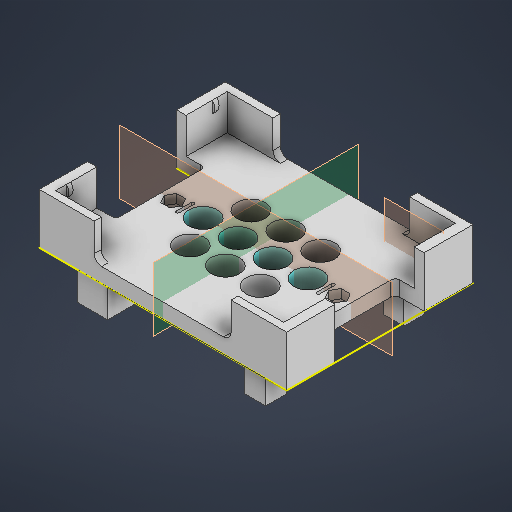
# Autodesk Inventor part: PILLARSCELLCASE18650
Saved by Autodesk Inventor 2026.2 (Build 302298000, 298)
## iProperties
Created: 2024-11-21
Part Number: PILLARSCELLCASE18650
Material: Generic
Document SubType Name: Modeling
Designer: cbast
Density: 1 g/cm^3
Appearance: Default
Mass: 190.937 g
Surface Area: 666.623 cm^2
Volume: 190.937 cm^3
Author: cbast
## iProperties of the stored document BatteryCasev1_3DPrint.ipt
Created: 2025-01-30
Part Number: BatteryCasev1_3DPrint
Material: Generic
Document SubType Name: Modeling
Designer: cbast
Density: 1 g/cm^3
Appearance: Default
Author: cbast
Autodesk Inventor part; units mm, degrees
ref_plane "YZ Plane" through (0, 0, 0) normal (1, 0, 0) x (0, 1, 0)
ref_plane "XZ Plane" through (0, 0, 0) normal (0, 1, 0) x (-1, 0, 0)
ref_plane "XY Plane" through (0, 0, 0) normal (0, 0, 1) x (1, 0, 0)
sketch "Sketch1" plane through (0, 0, 0) normal (0, 1, 0) x (-1, 0, 0)
  circle A0 centre (0, 0) radius 9.5
  circle A1 centre (23.5, 0) radius 9.5
  circle A2 centre (-23.5, 0) radius 9.5
  circle A3 centre (47, 0) radius 9.5
  line L0 (0, 0) -> (-32.9562, 0) construction
  line L1 (-32.9562, 0) -> (61.076, 0) construction
  circle A4 centre (0, 0) radius 14 construction
  circle A5 centre (-23.5, 0) radius 14 construction
  circle A6 centre (47, 0) radius 14 construction
  circle A7 centre (23.5, 0) radius 14 construction
  circle A8 centre (47, 0) radius 15 construction
  circle A9 centre (-23.5, 0) radius 15 construction
  circle A10 centre (0, 0) radius 15 construction
  circle A11 centre (23.5, 0) radius 15 construction
  line L2 (37.5, 0) -> (33, 0) construction
  circle A12 centre (35.25, -20.3516) radius 9.5
  circle A13 centre (35.25, -20.3516) radius 14 construction
  circle A14 centre (35.25, -20.3516) radius 15 construction
  line L3 (14, 0) -> (9.5, 0) construction
  line L4 (-9.5, 0) -> (-14, 0) construction
  line L5 (35.25, -20.3516) -> (-11.75, -20.3516) construction
  circle A15 centre (11.75, -20.3516) radius 9.5
  circle A16 centre (-11.75, -20.3516) radius 9.5
  circle A17 centre (11.75, -20.3516) radius 14 construction
  circle A18 centre (11.75, -20.3516) radius 15 construction
  circle A19 centre (-11.75, -20.3516) radius 14 construction
  circle A20 centre (-11.75, -20.3516) radius 15 construction
  circle A21 centre (35.25, 20.3516) radius 9.5
  circle A22 centre (35.25, 20.3516) radius 14 construction
  circle A23 centre (35.25, 20.3516) radius 15 construction
  line L6 (35.25, 20.3516) -> (-11.75, 20.3516) construction
  circle A24 centre (11.75, 20.3516) radius 9.5
  circle A25 centre (-11.75, 20.3516) radius 9.5
  circle A26 centre (11.75, 20.3516) radius 14 construction
  circle A27 centre (11.75, 20.3516) radius 15 construction
  circle A28 centre (-11.75, 20.3516) radius 14 construction
  circle A29 centre (-11.75, 20.3516) radius 15 construction
  arc A30 (49.1998, -14.8378) -> (49.1998, 14.8378) centre (47, 0) ccw
  arc A31 (49.1998, 14.8378) -> (23.5, 29.6756) centre (35.25, 20.3516) ccw
  arc A32 (23.5, 29.6756) -> (0, 29.6756) centre (11.75, 20.3516) ccw
  arc A33 (0, 29.6756) -> (-25.6998, 14.8378) centre (-11.75, 20.3516) ccw
  arc A34 (-25.6998, 14.8378) -> (-25.6998, -14.8378) centre (-23.5, 0) ccw
  arc A35 (-25.6998, -14.8378) -> (0, -29.6756) centre (-11.75, -20.3516) ccw
  arc A36 (0, -29.6756) -> (23.5, -29.6756) centre (11.75, -20.3516) ccw
  arc A37 (23.5, -29.6756) -> (49.1998, -14.8378) centre (35.25, -20.3516) ccw
  point P0 (46.8931, -14.9996)
  point P1 (46.8931, 14.9996)
  point P2 (-23.3931, 14.9996)
  point P3 (-23.3931, -14.9996)
  dimension "d145" = 28
  dimension "d149" = 28
  dimension "d0" = 19
  dimension "d2" = 19
  dimension "d4" = 19
  dimension "d53" = 19
  dimension "d144" = 28
  dimension "d150" = 28
  dimension "d154" = 30
  dimension "d158" = 30
  dimension "d162" = 30
  dimension "d163" = 30
  dimension "d291" = 19
  dimension "d292" = 28
  dimension "d293" = 30
  dimension "d294" = 19
  dimension "d295" = 19
  dimension "d296" = 28
  dimension "d297" = 30
  dimension "d298" = 28
  dimension "d299" = 30
  constraints: 40 point on circle, 36 centre point, 32 coincident, 12 end point, 10 vertical alignment, 9 equal radius, 4 tangent, 2 horizontal alignment, 1 horizontal, 1 midpoint, 1 parallel, 1 point on line, 17 other
  measures "d0" diameter of A0
  measures "d2" diameter of A1
  measures "d4" diameter of A2
  measures "d53" diameter of A3
  measures "d144" diameter of A4
  measures "d150" diameter of A7
  measures "d154" diameter of A8
  measures "d158" diameter of A9
  measures "d162" diameter of A10
  measures "d163" diameter of A11
  measures "d291" diameter of A12
  measures "d292" diameter of A13
  measures "d293" diameter of A14
  measures "d294" diameter of A15
  measures "d295" diameter of A16
  measures "d296" diameter of A17
  measures "d297" diameter of A18
  measures "d298" diameter of A19
  measures "d299" diameter of A20
extrude "Extrusion1" add sketch "Sketch1" along normal blind 15
sketch "Sketch26" plane through (0, 15, 0) normal (0, 1, 0) x (1, 0, 0)
  arc A0 (-49.1998, -14.8378) -> (-23.5, -29.6756) centre (-35.25, -20.3516) ccw projected
  arc A1 (-23.5, -29.6756) -> (0, -29.6756) centre (-11.75, -20.3516) ccw projected
  arc A2 (0, -29.6756) -> (25.6998, -14.8378) centre (11.75, -20.3516) ccw projected
  arc A3 (25.6998, -14.8378) -> (25.6998, 14.8378) centre (23.5, 0) ccw projected
  arc A4 (25.6998, 14.8378) -> (0, 29.6756) centre (11.75, 20.3516) ccw projected
  arc A5 (0, 29.6756) -> (-23.5, 29.6756) centre (-11.75, 20.3516) ccw projected
  arc A6 (-23.5, 29.6756) -> (-49.1998, 14.8378) centre (-35.25, 20.3516) ccw projected
  arc A7 (-49.1998, 14.8378) -> (-49.1998, -14.8378) centre (-47, 0) ccw projected
  circle A8 centre (0, 0) radius 9.5 projected
  circle A9 centre (-23.5, 0) radius 9.5 projected
  circle A10 centre (11.75, -20.3516) radius 9.5 projected
  circle A11 centre (-11.75, -20.3516) radius 9.5 projected
  circle A12 centre (-35.25, -20.3516) radius 9.5 projected
  circle A13 centre (11.75, 20.3516) radius 9.5 projected
  circle A14 centre (-11.75, 20.3516) radius 9.5 projected
  circle A15 centre (-35.25, 20.3516) radius 9.5 projected
  circle A16 centre (-47, 0) radius 9.5 projected
  circle A17 centre (23.5, 0) radius 9.5 projected
  line L0 (-88.45, 57.7) -> (64.95, 57.7)
  line L1 (64.95, 57.7) -> (64.95, -57.7)
  line L2 (64.95, -57.7) -> (-88.45, -57.7)
  line L3 (-88.45, -57.7) -> (-88.45, 57.7)
  line L4 (-88.45, 57.7) -> (64.95, -57.7) construction
  line L5 (64.95, 57.7) -> (-88.45, -57.7) construction
  line L6 (-88.45, 0) -> (-62, 0) construction
  line L7 (38.5, 0) -> (64.95, 0) construction
  point P0 (-11.75, 0)
  dimension "d300" = 153.4
  dimension "d301" = 115.4
  constraints: 16 end point, 4 midpoint, 3 equal length, 2 horizontal, 2 point on circle, 1 collinear, 1 perpendicular
  measures "d300" distance of L1.end L2.end
  measures "d301" distance of L0.end L1.end
extrude "Extrusion24" add sketch "Sketch26" against normal blind 10 contours L0 L1 L2 L3
sketch "Sketch28" plane through (0, 15, 0) normal (0, 1, 0) x (1, 0, 0)
  line L0 (-88.45, -57.7) -> (64.95, -57.7) projected
  line L1 (64.95, -57.7) -> (64.95, 57.7) projected
  line L2 (64.95, 57.7) -> (-88.45, 57.7) projected
  line L3 (-88.45, 57.7) -> (-88.45, -57.7) projected
  circle A0 centre (0, 0) radius 9.5 projected
  circle A1 centre (-23.5, 0) radius 9.5 projected
  circle A2 centre (11.75, -20.3516) radius 9.5 projected
  circle A3 centre (-11.75, -20.3516) radius 9.5 projected
  circle A4 centre (-35.25, -20.3516) radius 9.5 projected
  circle A5 centre (11.75, 20.3516) radius 9.5 projected
  circle A6 centre (-11.75, 20.3516) radius 9.5 projected
  circle A7 centre (-35.25, 20.3516) radius 9.5 projected
  circle A8 centre (-47, 0) radius 9.5 projected
  circle A9 centre (23.5, 0) radius 9.5 projected
  line L4 (64.95, 57.7) -> (64.95, -57.7) projected
  line L5 (-88.0641, -57.4308) -> (64.95, -57.4308)
  line L6 (64.95, -57.4308) -> (64.95, 57.7)
  line L7 (64.95, 57.7) -> (-88.0641, 57.7)
  line L8 (-88.0641, 57.7) -> (-88.0641, -57.4308)
  line L9 (-88.0641, -57.4308) -> (64.95, 57.7) construction
  line L10 (64.95, -57.4308) -> (-88.0641, 57.7) construction
  line L11 (-94.7093, -62.4308) -> (71.5952, -62.4308)
  line L12 (71.5952, -62.4308) -> (71.5952, 62.7)
  line L13 (71.5952, 62.7) -> (-94.7093, 62.7)
  line L14 (-94.7093, 62.7) -> (-94.7093, -62.4308)
  line L15 (-94.7093, -62.4308) -> (71.5952, 62.7) construction
  line L16 (71.5952, -62.4308) -> (-94.7093, 62.7) construction
  point P0 (-11.5571, 0.1346)
  point P1 (-11.5571, 0.1346)
  dimension "d306" = 5
  constraints: 24 end point, 5 midpoint, 4 parallel, 2 horizontal, 2 perpendicular, 1 point on line
  measures "d306" distance between parallel lines of L13 L2
extrude "Extrusion25" add sketch "Sketch28" along normal blind 24 and the other way blind 10 contours L14 L13 L12 L11
sketch "Sketch29" plane through (-94.7093, 39, 62.4308) normal (0, 0, 1) x (1, 0, 0)
  line L0 (6.2593, -24) -> (159.6593, -24) projected
  line L1 (41.9593, -24) -> (123.9593, -24)
  line L2 (166.3046, 0) -> (0, 0) projected
  line L3 (128.9593, -24) -> (36.9593, -24)
  line L4 (36.9593, -19) -> (36.9593, 0)
  line L5 (36.9593, 0) -> (128.9593, 0)
  line L6 (128.9593, 0) -> (128.9593, -19)
  arc A0 (36.9593, -19) -> (41.9593, -24) centre (41.9593, -19) ccw
  arc A1 (123.9593, -24) -> (128.9593, -19) centre (123.9593, -19) ccw
  point P0 (94.7093, -39)
  point P1 (82.9593, -24)
  point P2 (42.9593, -24)
  point P3 (128.9593, 0)
  dimension "d311" = 86
  dimension "d312" = 5
  constraints: 10 end point, 6 point on line, 4 point on circle, 4 tangent, 2 centre point, 2 midpoint, 2 parallel, 1 equal radius, 1 horizontal, 1 perpendicular
  measures "d311" distance of point (42.959, -24) L3.start
  measures "d312" radius of A0
extrude "Extrusion26" cut sketch "Sketch29" against normal through all
sketch "Sketch30" plane through (0, 39, 0) normal (0, 1, 0) x (1, 0, 0)
  circle A0 centre (-47, 0) radius 9.5 projected
  circle A1 centre (0, 0) radius 9.5 projected
  circle A2 centre (-23.5, 0) radius 9.5 projected
  circle A3 centre (11.75, -20.3516) radius 9.5 projected
  circle A4 centre (-11.75, -20.3516) radius 9.5 projected
  circle A5 centre (-35.25, -20.3516) radius 9.5 projected
  circle A6 centre (11.75, 20.3516) radius 9.5 projected
  circle A7 centre (-11.75, 20.3516) radius 9.5 projected
  circle A8 centre (-35.25, 20.3516) radius 9.5 projected
  circle A9 centre (23.5, 0) radius 9.5 projected
  line L0 (29.25, -57.7) -> (64.95, -57.7) projected
  line L1 (64.95, -57.7) -> (64.95, 57.7) projected
  line L2 (64.95, 57.7) -> (29.25, 57.7) projected
  line L3 (29.25, 57.7) -> (29.25, 62.7) projected
  line L4 (-52.75, 62.7) -> (29.25, 62.7) projected
  line L5 (-52.75, 57.7) -> (-52.75, 62.7) projected
  line L6 (-52.75, 57.7) -> (-88.45, 57.7) projected
  line L7 (-88.45, 57.7) -> (-88.45, -57.7) projected
  line L8 (-88.45, -57.7) -> (-52.75, -57.7) projected
  line L9 (-52.75, -62.4308) -> (-52.75, -57.7) projected
  line L10 (29.25, -62.4308) -> (-52.75, -62.4308) projected
  line L11 (29.25, -62.4308) -> (29.25, -57.7) projected
  line L12 (34.25, -57.7) -> (34.25, -62.4308) projected
  line L13 (34.25, -62.4308) -> (71.5952, -62.4308) projected
  line L14 (71.5952, -62.4308) -> (71.5952, 62.7) projected
  line L15 (71.5952, 62.7) -> (34.25, 62.7) projected
  line L16 (34.25, 62.7) -> (34.25, 57.7) projected
  line L17 (34.25, 57.7) -> (64.95, 57.7) projected
  line L18 (64.95, 57.7) -> (64.95, -57.7) projected
  line L19 (64.95, -57.7) -> (34.25, -57.7) projected
  line L20 (-88.45, -57.7) -> (-88.45, 57.7) projected
  line L21 (-57.75, -62.4308) -> (-57.75, -57.7) projected
  line L22 (-57.75, -57.7) -> (-88.45, -57.7) projected
  line L23 (-88.45, -57.7) -> (-88.45, 57.7) projected
  line L24 (-88.45, 57.7) -> (-57.75, 57.7) projected
  line L25 (-57.75, 57.7) -> (-57.75, 62.7) projected
  line L26 (-57.75, 62.7) -> (-94.7093, 62.7) projected
  line L27 (-94.7093, 62.7) -> (-94.7093, -62.4308) projected
  line L28 (-94.7093, -62.4308) -> (-57.75, -62.4308) projected
  line L29 (-88.45, -30) -> (-88.45, 30)
  line L30 (-94.7093, -62.4308) -> (-94.7093, 62.7) projected
  line L31 (-75.7093, 27) -> (-75.7093, -27)
  arc A10 (-75.7093, 27) -> (-78.7093, 30) centre (-78.7093, 27) ccw
  arc A11 (-78.7093, -30) -> (-75.7093, -27) centre (-78.7093, -27) ccw
  line L32 (-94.7093, 0) -> (-47, 0) construction
  line L33 (-47, 0) -> (-94.7093, 0) construction
  line L34 (-78.7093, 30) -> (-114.521, 30)
  line L35 (-114.521, 30) -> (-114.521, -30)
  line L36 (-114.521, -30) -> (-78.7093, -30)
  point P0 (-88.45, 0)
  dimension "d317" = 3
  constraints: 14 end point, 4 point on circle, 3 perpendicular, 2 centre point, 2 midpoint, 2 tangent, 1 collinear, 1 equal radius, 1 horizontal
  measures "d317" radius of A10
extrude "Extrusion27" cut sketch "Sketch30" against normal through all contours L36 L27 L34 L7 | L7 L34 A10 L31 A11 L36 | L36 L35 L34 L27
ref_plane "Work Plane9" through (-11.75, 15, -57.7) normal (-1, 0, 0) x (0, 0, 1)
sketch "Sketch31" plane through (0, 15, 0) normal (0, 1, 0) x (1, 0, 0)
  line L0 (-64.06, 5.3) -> (-61, 0)
  line L1 (-61, 0) -> (-64.06, -5.3)
  line L2 (-64.06, -5.3) -> (-70.1799, -5.3)
  line L3 (-70.1799, -5.3) -> (-73.2398, 0)
  line L4 (-73.2398, 0) -> (-70.1799, 5.3)
  line L5 (-70.1799, 5.3) -> (-64.06, 5.3)
  line L6 (-88.45, 57.7) -> (-57.75, 57.7) projected
  circle A0 centre (-47, 0) radius 9.5 projected
  line L7 (-57.75, -57.7) -> (-88.45, -57.7) projected
  line L8 (-75.7093, -27) -> (-75.7093, 27) construction
  line L9 (-75.7093, 0) -> (-47, 0) construction
  point P0 (0, 0)
  point P1 (-67.1199, 0)
  dimension "d323" = 14
  dimension "d332" = 10.6
  constraints: 14 end point, 2 parallel, 1 midpoint, 1 perpendicular, 1 point on line, 13 other
  measures "d323" distance of L9.end L0.end
  measures "d332" distance between parallel lines of L2 L5
extrude "Extrusion28" cut sketch "Sketch31" against normal blind 6 contours L0 L1 L2 L3 L4 L5
sketch "Sketch32" plane through (0, 9, 0) normal (0, 1, 0) x (1, 0, 0)
  line L0 (-73.2398, 0) -> (-70.1799, 5.3) projected
  line L1 (-70.1799, -5.3) -> (-73.2398, 0) projected
  line L2 (-64.06, -5.3) -> (-70.1799, -5.3) projected
  line L3 (-61, 0) -> (-64.06, -5.3) projected
  line L4 (-64.06, 5.3) -> (-61, 0) projected
  line L5 (-70.1799, 5.3) -> (-64.06, 5.3) projected
  circle A0 centre (-67.1199, 0) radius 3.25
  line L6 (-63.8699, 0) -> (-61, 0) construction
  line L7 (-70.3699, 0) -> (-73.2398, 0) construction
  point P0 (0, 0)
  dimension "d329" = 6.5
  constraints: 4 end point, 2 collinear, 2 point on circle, 1 centre point, 1 horizontal, 1 point on line
  measures "d329" diameter of A0
extrude "Extrusion29" cut sketch "Sketch32" against normal through all contours A0
sketch "Sketch33" plane through (0, 15, 0) normal (0, 1, 0) x (1, 0, 0)
  line L0 (-70.1799, -5.3) -> (-73.2398, 0) projected
  line L1 (-73.2398, 0) -> (-70.1799, 5.3) projected
  line L2 (-70.1799, 5.3) -> (-64.06, 5.3) projected
  line L3 (-64.06, 5.3) -> (-61, 0) projected
  line L4 (-61, 0) -> (-64.06, -5.3) projected
  line L5 (-64.06, -5.3) -> (-70.1799, -5.3) projected
  circle A0 centre (23.5, 0) radius 9.5 projected
  circle A1 centre (-35.25, 20.3516) radius 9.5 projected
  circle A2 centre (-11.75, 20.3516) radius 9.5 projected
  circle A3 centre (11.75, 20.3516) radius 9.5 projected
  circle A4 centre (-35.25, -20.3516) radius 9.5 projected
  circle A5 centre (-11.75, -20.3516) radius 9.5 projected
  circle A6 centre (11.75, -20.3516) radius 9.5 projected
  circle A7 centre (-23.5, 0) radius 9.5 projected
  circle A8 centre (0, 0) radius 9.5 projected
  circle A9 centre (-47, 0) radius 9.5 projected
  line L6 (64.95, -57.7) -> (64.95, 57.7) projected
  line L7 (64.95, 57.7) -> (29.25, 57.7) projected
  line L8 (29.25, 57.7) -> (29.25, 62.7) projected
  line L9 (-52.75, 62.7) -> (29.25, 62.7) projected
  line L10 (-52.75, 57.7) -> (-52.75, 62.7) projected
  line L11 (-52.75, 57.7) -> (-88.45, 57.7) projected
  line L12 (-88.45, 57.7) -> (-88.45, 30) projected
  line L13 (-88.45, -57.7) -> (-52.75, -57.7) projected
  line L14 (-52.75, -62.4308) -> (-52.75, -57.7) projected
  line L15 (29.25, -62.4308) -> (-52.75, -62.4308) projected
  line L16 (29.25, -62.4308) -> (29.25, -57.7) projected
  line L17 (29.25, -57.7) -> (64.95, -57.7) projected
  line L18 (-59, 6) -> (-59, -6) construction
  line L19 (-60, 5) -> (-60, -5)
  line L20 (-58, -5) -> (-58, 5)
  arc A10 (-58, 5) -> (-60, 5) centre (-59, 5) ccw
  arc A11 (-60, -5) -> (-58, -5) centre (-59, -5) ccw
  line L21 (-47, 0) -> (-75.7093, 0) construction
  line L22 (-88.45, 30) -> (-78.7093, 30) projected
  arc A12 (-75.7093, 27) -> (-78.7093, 30) centre (-78.7093, 27) ccw projected
  line L23 (-75.7093, 27) -> (-75.7093, -27) projected
  arc A13 (-78.7093, -30) -> (-75.7093, -27) centre (-78.7093, -27) ccw projected
  line L24 (-78.7093, -30) -> (-88.45, -30) projected
  line L25 (-88.45, -30) -> (-88.45, -57.7) projected
  point P0 (-59, 0)
  dimension "d333" = 12
  dimension "d334" = 2
  dimension "d335" = 11
  constraints: 10 end point, 6 point on circle, 4 tangent, 3 point on line, 2 centre point, 1 midpoint, 1 parallel, 1 vertical
  measures "d333" distance of L18.start L18.end
  measures "d334" diameter of A11
  measures "d335" distance from line of L20 L21.start
extrude "Extrusion30" cut sketch "Sketch33" against normal through all contours A10 L20 A11 L19
mirror "Mirror9" about plane through (-11.75, 15, -57.7) normal (-1, 0, 0) of "Extrusion28", "Extrusion29", "Extrusion30"
ref_plane "Work Plane10" through (-94.7093, 5, -0.1346) normal (0, 0, 1) x (1, 0, 0)
ref_plane "Work Plane11" through (64.95, 15, -47.7) normal (0, 0, 1) x (1, 0, 0)
sketch "Sketch34" plane through (64.95, 15, -47.7) normal (0, 0, 1) x (1, 0, 0)
  line L0 (0, 24) -> (0, 0) projected
  line L1 (0, 0) -> (0, 16) construction
  line L2 (0, 0) -> (0, 24) construction
  line L3 (0, 16) -> (0, 24)
  arc A0 (0, 24) -> (0, 16) centre (0, 20) ccw
  arc A1 (0, 24) -> (0, 16) centre (4.4721, 20) ccw
  point P0 (-64.95, -15)
  dimension "d339" = 16
  dimension "d340" = 8
  dimension "d342" = 6
  constraints: 4 end point, 4 point on circle, 2 centre point, 2 point on line
  measures "d339" distance of L0.end L1.end
  measures "d340" distance of L1.end L3.end
  measures "d342" radius of A1
extrude "Extrusion31" add sketch "Sketch34" against normal blind 3 contours L0 A1
mirror "Mirror10" about plane through (-11.75, 15, -57.7) normal (-1, 0, 0) of "Extrusion31"
mirror "Mirror11" about plane through (-94.7093, 5, -0.1346) normal (0, 0, 1) of "Extrusion31", "Mirror10"
sketch "Sketch35" plane through (0, 5, 0) normal (0, -1, 0) x (1, 0, 0)
  line L0 (-94.7093, -62.7) -> (71.5952, -62.7) projected
  circle A0 centre (43.6199, 0) radius 3.25 projected
  circle A1 centre (-67.1199, 0) radius 3.25 projected
  arc A2 (-49.1998, 14.8378) -> (-49.1998, -14.8378) centre (-47, 0) ccw projected
  arc A3 (-23.5, 29.6756) -> (-49.1998, 14.8378) centre (-35.25, 20.3516) ccw projected
  arc A4 (0, 29.6756) -> (-23.5, 29.6756) centre (-11.75, 20.3516) ccw projected
  arc A5 (25.6998, 14.8378) -> (0, 29.6756) centre (11.75, 20.3516) ccw projected
  arc A6 (25.6998, -14.8378) -> (25.6998, 14.8378) centre (23.5, 0) ccw projected
  arc A7 (0, -29.6756) -> (25.6998, -14.8378) centre (11.75, -20.3516) ccw projected
  arc A8 (-23.5, -29.6756) -> (0, -29.6756) centre (-11.75, -20.3516) ccw projected
  arc A9 (-49.1998, -14.8378) -> (-23.5, -29.6756) centre (-35.25, -20.3516) ccw projected
  line L1 (-94.7093, -30) -> (-94.7093, -62.7) projected
  line L2 (-94.7093, -62.7) -> (71.5952, -62.7) projected
  line L3 (71.5952, -62.7) -> (71.5952, 62.4308) projected
  line L4 (71.5952, 62.4308) -> (-94.7093, 62.4308) projected
  line L5 (-78.7093, -30) -> (-94.7093, -30) projected
  line L6 (-94.7093, 62.4308) -> (-94.7093, 30) projected
  line L7 (-94.7093, 30) -> (-78.7093, 30) projected
  arc A10 (-75.7093, 27) -> (-78.7093, 30) centre (-78.7093, 27) ccw projected
  line L8 (-75.7093, 27) -> (-75.7093, -27) projected
  arc A11 (-78.7093, -30) -> (-75.7093, -27) centre (-78.7093, -27) ccw projected
  point P0 (0, 0)
sketch "Sketch36" plane through (0, 15, 0) normal (0, 1, 0) x (1, 0, 0)
  line L0 (-88.45, 30) -> (-78.7093, 30) construction
  line L1 (-78.7093, -30) -> (-88.45, -30) construction
  line L2 (-75.7093, 27) -> (-75.7093, -27) construction
  line L3 (64.95, 47.7) -> (64.95, -47.4308) construction
  line L4 (71.5952, 62.7) -> (71.5952, -62.4308) construction
  line L5 (64.95, 20.5623) -> (52.209, 20.5623) construction
  line L6 (-75.7093, -2.0148) -> (-75.7093, -47.4308) construction
  line L7 (52.24, 27) -> (52.24, -27)
  line L8 (55.24, -30) -> (114.3089, -30)
  line L9 (114.3089, -30) -> (114.3089, 30)
  line L10 (114.3089, 30) -> (55.24, 30)
  arc A0 (55.24, 30) -> (52.24, 27) centre (55.24, 27) ccw
  arc A1 (52.24, -27) -> (55.24, -30) centre (55.24, -27) ccw
  point P0 (0, 0)
  dimension "d347" = 12.741
  dimension "d348" = 3
  constraints: 12 end point, 4 point on circle, 4 tangent, 3 perpendicular, 3 point on line, 2 centre point, 1 equal radius, 1 horizontal, 1 vertical
  measures "d347" distance of L5.start L5.end
  measures "d348" radius of A0
extrude "Extrusion32" cut sketch "Sketch36" along normal through all both and the other way through all
sketch "Sketch37" plane through (0, 5, 0) normal (0, -1, 0) x (1, 0, 0)
  line L0 (-72.2093, 38.9308) -> (-57.2093, 38.9308)
  line L1 (-57.2093, 38.9308) -> (-57.2093, 53.9308)
  line L2 (-57.2093, 53.9308) -> (-72.2093, 53.9308)
  line L3 (-72.2093, 53.9308) -> (-72.2093, 38.9308)
  line L4 (-72.2093, 38.9308) -> (-57.2093, 53.9308) construction
  line L5 (-57.2093, 38.9308) -> (-72.2093, 53.9308) construction
  line L6 (-74.7093, 36.4308) -> (-54.7093, 36.4308)
  line L7 (-54.7093, 36.4308) -> (-54.7093, 56.4308)
  line L8 (-54.7093, 56.4308) -> (-74.7093, 56.4308)
  line L9 (-74.7093, 56.4308) -> (-74.7093, 36.4308)
  line L10 (-74.7093, 36.4308) -> (-54.7093, 56.4308) construction
  line L11 (-54.7093, 36.4308) -> (-74.7093, 56.4308) construction
  line L12 (-94.7093, 62.4308) -> (-94.7093, 30) projected
  line L13 (71.5952, 62.4308) -> (-94.7093, 62.4308) projected
  line L14 (34.5952, 39.4308) -> (48.5952, 39.4308)
  line L15 (48.5952, 39.4308) -> (48.5952, 53.4308)
  line L16 (48.5952, 53.4308) -> (34.5952, 53.4308)
  line L17 (34.5952, 53.4308) -> (34.5952, 39.4308)
  line L18 (34.5952, 39.4308) -> (48.5952, 53.4308) construction
  line L19 (48.5952, 39.4308) -> (34.5952, 53.4308) construction
  line L20 (71.5952, 30) -> (71.5952, 62.4308) projected
  line L21 (-75.7093, -27) -> (-75.7093, 27) construction
  line L22 (-75.7093, 0) -> (52.24, 0) construction
  line L23 (52.24, -27) -> (52.24, 27) construction
  line L24 (-72.2093, -38.9308) -> (-57.2093, -38.9308)
  line L25 (-57.2093, -38.9308) -> (-57.2093, -53.9308)
  line L26 (-57.2093, -53.9308) -> (-72.2093, -53.9308)
  line L27 (-72.2093, -53.9308) -> (-72.2093, -38.9308)
  line L28 (-72.2093, -38.9308) -> (-57.2093, -53.9308) construction
  line L29 (-57.2093, -38.9308) -> (-72.2093, -53.9308) construction
  line L30 (-74.7093, -36.4308) -> (-54.7093, -36.4308)
  line L31 (-54.7093, -36.4308) -> (-54.7093, -56.4308)
  line L32 (-54.7093, -56.4308) -> (-74.7093, -56.4308)
  line L33 (-74.7093, -56.4308) -> (-74.7093, -36.4308)
  line L34 (-74.7093, -36.4308) -> (-54.7093, -56.4308) construction
  line L35 (-54.7093, -36.4308) -> (-74.7093, -56.4308) construction
  line L36 (34.5952, -39.4308) -> (48.5952, -39.4308)
  line L37 (48.5952, -39.4308) -> (48.5952, -53.4308)
  line L38 (48.5952, -53.4308) -> (34.5952, -53.4308)
  line L39 (34.5952, -53.4308) -> (34.5952, -39.4308)
  line L40 (34.5952, -39.4308) -> (48.5952, -53.4308) construction
  line L41 (48.5952, -39.4308) -> (34.5952, -53.4308) construction
  point P0 (0, 0)
  point P1 (-64.7093, 46.4308)
  point P2 (41.5952, 46.4308)
  point P3 (-64.7093, -46.4308)
  point P4 (41.5952, -46.4308)
  dimension "d351" = 15
  dimension "d352" = 20
  dimension "d355" = 16
  dimension "d356" = 30
  dimension "d357" = 14
  dimension "d358" = 14
  dimension "d359" = 16
  dimension "d360" = 30
  constraints: 74 end point, 14 symmetric about line, 8 midpoint, 6 parallel, 4 perpendicular, 3 horizontal, 2 point on line
  measures "d351" distance of L2.end L0.start
  measures "d352" distance of L8.end L6.start
  measures "d355" distance from line of L13 point (-64.709, 46.431)
  measures "d356" distance from line of point (-64.709, 46.431) L12
  measures "d357" distance of L15.end L16.end
  measures "d358" distance of L16.end L14.start
  measures "d359" distance from line of point (41.595, 46.431) L13
  measures "d360" distance from line of L20 point (41.595, 46.431)
extrude "Extrusion33" add sketch "Sketch37" along normal blind 25
sketch "Sketch38" plane through (0, 5, 0) normal (0, -1, 0) x (1, 0, 0)
  line L0 (-72.2093, 38.9308) -> (-57.2093, 38.9308) projected
  line L1 (-57.2093, 38.9308) -> (-57.2093, 53.9308) projected
  line L2 (-57.2093, 53.9308) -> (-72.2093, 53.9308) projected
  line L3 (-72.2093, 53.9308) -> (-72.2093, 38.9308) projected
  line L4 (-57.2093, -53.9308) -> (-57.2093, -38.9308) projected
  line L5 (-57.2093, -38.9308) -> (-72.2093, -38.9308) projected
  line L6 (-72.2093, -38.9308) -> (-72.2093, -53.9308) projected
  line L7 (-72.2093, -53.9308) -> (-57.2093, -53.9308) projected
  line L8 (-72.2093, 53.9308) -> (-57.2093, 53.9308)
  line L9 (-57.2093, 53.9308) -> (-57.2093, 38.9308)
  line L10 (-57.2093, 38.9308) -> (-72.2093, 38.9308)
  line L11 (-72.2093, 38.9308) -> (-72.2093, 53.9308)
  line L12 (-72.2093, -38.9308) -> (-57.2093, -38.9308)
  line L13 (-57.2093, -38.9308) -> (-57.2093, -53.9308)
  line L14 (-57.2093, -53.9308) -> (-72.2093, -53.9308)
  line L15 (-72.2093, -53.9308) -> (-72.2093, -38.9308)
  point P0 (0, 0)
  constraints: 16 end point, 4 parallel, 2 horizontal, 2 perpendicular
extrude "Extrusion34" add sketch "Sketch38" along normal blind 12.5
sketch "Sketch39" plane through (0, 5, 0) normal (0, -1, 0) x (1, 0, 0)
  line L0 (-23.519, 56.6377) -> (0.6762, 56.6377) construction
  line L1 (0.6762, 56.6377) -> (0.6762, 41.0836) construction
  line L2 (0.6762, 41.0836) -> (-23.519, 41.0836) construction
  line L3 (-23.519, 41.0836) -> (-23.519, 56.6377) construction
  line L4 (-21.6935, 53.5333) -> (-20.6628, 56.5833)
  line L5 (-20.6628, 56.5833) -> (-19.8274, 56.5833)
  line L6 (-19.8274, 56.5833) -> (-18.7967, 53.5333)
  line L7 (-18.7967, 53.5333) -> (-19.5852, 53.5333)
  line L8 (-19.5852, 53.5333) -> (-19.7755, 54.1561)
  line L9 (-19.7755, 54.1561) -> (-20.7345, 54.1561)
  line L10 (-20.7345, 54.1561) -> (-20.9273, 53.5333)
  line L11 (-20.9273, 53.5333) -> (-21.6935, 53.5333)
  line L12 (-19.9436, 54.7098) -> (-20.255, 55.7182)
  line L13 (-20.255, 55.7182) -> (-20.5689, 54.7098)
  line L14 (-20.5689, 54.7098) -> (-19.9436, 54.7098)
  line L15 (-15.6751, 53.5333) -> (-16.6069, 53.5333)
  line L16 (-16.6069, 53.5333) -> (-17.4546, 54.6529)
  line L17 (-17.4546, 54.6529) -> (-17.7315, 54.6529)
  line L18 (-17.7315, 54.6529) -> (-17.7315, 53.5333)
  line L19 (-17.7315, 53.5333) -> (-18.4927, 53.5333)
  line L20 (-18.4927, 53.5333) -> (-18.4927, 56.5833)
  line L21 (-18.4927, 56.5833) -> (-17.2668, 56.5833)
  spline S0 degree 2 poles (-17.2668, 56.5833) (-17.0122, 56.5833) (-16.6365, 56.519) (-16.4759, 56.4201) knots 0 0 0 1 2 2 2
  spline S1 degree 2 poles (-16.4759, 56.4201) (-16.3127, 56.3163) (-16.12, 55.9926) (-16.12, 55.7454) knots 0 0 0 1 2 2 2
  spline S2 degree 2 poles (-16.12, 55.7454) (-16.12, 55.3969) (-16.4363, 54.9594) (-16.7008, 54.8309) knots 0 0 0 1 2 2 2
  line L22 (-16.7008, 54.8309) -> (-15.6751, 53.5333)
  spline S3 degree 2 poles (-16.9059, 55.649) (-16.9059, 55.7652) (-16.9949, 55.9308) (-17.0963, 55.9753) knots 0 0 0 1 2 2 2
  spline S4 degree 2 poles (-17.0963, 55.9753) (-17.1679, 56.0049) (-17.3434, 56.0222) (-17.4744, 56.0222) knots 0 0 0 1 2 2 2
  line L23 (-17.4744, 56.0222) -> (-17.7315, 56.0222)
  line L24 (-17.7315, 56.0222) -> (-17.7315, 55.2016)
  line L25 (-17.7315, 55.2016) -> (-17.5115, 55.2016)
  spline S5 degree 2 poles (-17.5115, 55.2016) (-17.3533, 55.2016) (-17.1284, 55.2412) (-17.0518, 55.303) knots 0 0 0 1 2 2 2
  spline S6 degree 2 poles (-17.0518, 55.303) (-16.9776, 55.3623) (-16.9059, 55.5205) (-16.9059, 55.649) knots 0 0 0 1 2 2 2
  line L26 (-14.8619, 53.5333) -> (-14.8619, 56.0024)
  line L27 (-14.8619, 56.0024) -> (-15.764, 56.0024)
  line L28 (-15.764, 56.0024) -> (-15.764, 56.5833)
  line L29 (-15.764, 56.5833) -> (-13.1935, 56.5833)
  line L30 (-13.1935, 56.5833) -> (-13.1935, 56.0024)
  line L31 (-13.1935, 56.0024) -> (-14.0957, 56.0024)
  line L32 (-14.0957, 56.0024) -> (-14.0957, 53.5333)
  line L33 (-14.0957, 53.5333) -> (-14.8619, 53.5333)
  spline S7 degree 2 poles (-11.938, 53.4789) (-12.2889, 53.4789) (-12.8179, 53.6148) (-13.0452, 53.7137) knots 0 0 0 1 2 2 2
  line L34 (-13.0452, 53.7137) -> (-13.0452, 54.4404)
  line L35 (-13.0452, 54.4404) -> (-12.976, 54.4404)
  spline S8 degree 2 poles (-12.976, 54.4404) (-12.7462, 54.2451) (-12.195, 54.035) (-11.9355, 54.035) knots 0 0 0 1 2 2 2
  spline S9 degree 2 poles (-11.9355, 54.035) (-11.8687, 54.035) (-11.6537, 54.0647) (-11.5894, 54.0943) knots 0 0 0 1 2 2 2
  spline S10 degree 2 poles (-11.5894, 54.0943) (-11.5104, 54.1289) (-11.3991, 54.255) (-11.3991, 54.3563) knots 0 0 0 1 2 2 2
  spline S11 degree 2 poles (-11.3991, 54.3563) (-11.3991, 54.4725) (-11.5796, 54.6159) (-11.7031, 54.648) knots 0 0 0 1 2 2 2
  spline S12 degree 2 poles (-11.7031, 54.648) (-11.8589, 54.69) (-12.2123, 54.7617) (-12.368, 54.8161) knots 0 0 0 1 2 2 2
  spline S13 degree 2 poles (-12.368, 54.8161) (-12.7215, 54.9396) (-13.0279, 55.3623) (-13.0279, 55.6787) knots 0 0 0 1 2 2 2
  spline S14 degree 2 poles (-13.0279, 55.6787) (-13.0279, 56.1062) (-12.3038, 56.6377) (-11.76, 56.6377) knots 0 0 0 1 2 2 2
  spline S15 degree 2 poles (-11.76, 56.6377) (-11.4881, 56.6377) (-10.9493, 56.5264) (-10.7367, 56.4325) knots 0 0 0 1 2 2 2
  line L36 (-10.7367, 56.4325) -> (-10.7367, 55.7355)
  line L37 (-10.7367, 55.7355) -> (-10.8035, 55.7355)
  spline S16 degree 2 poles (-10.8035, 55.7355) (-10.974, 55.8813) (-11.4634, 56.0815) (-11.7204, 56.0815) knots 0 0 0 1 2 2 2
  spline S17 degree 2 poles (-11.7204, 56.0815) (-11.8218, 56.0815) (-11.98, 56.0519) (-12.0689, 56.0123) knots 0 0 0 1 2 2 2
  spline S18 degree 2 poles (-12.0689, 56.0123) (-12.1406, 55.9802) (-12.2444, 55.8517) (-12.2444, 55.7726) knots 0 0 0 1 2 2 2
  spline S19 degree 2 poles (-12.2444, 55.7726) (-12.2444, 55.6539) (-12.0788, 55.518) (-11.8416, 55.4636) knots 0 0 0 1 2 2 2
  spline S20 degree 2 poles (-11.8416, 55.4636) (-11.6883, 55.429) (-11.4041, 55.3623) (-11.2409, 55.3054) knots 0 0 0 1 2 2 2
  spline S21 degree 2 poles (-11.2409, 55.3054) (-10.9246, 55.1893) (-10.6156, 54.8037) (-10.6156, 54.4873) knots 0 0 0 1 2 2 2
  spline S22 degree 2 poles (-10.6156, 54.4873) (-10.6156, 54.0325) (-11.3299, 53.4789) (-11.938, 53.4789) knots 0 0 0 1 2 2 2
  line L38 (-6.9601, 53.5333) -> (-8.9942, 53.5333)
  line L39 (-8.9942, 53.5333) -> (-8.9942, 56.5833)
  line L40 (-8.9942, 56.5833) -> (-8.228, 56.5833)
  line L41 (-8.228, 56.5833) -> (-8.228, 54.1141)
  line L42 (-8.228, 54.1141) -> (-6.9601, 54.1141)
  line L43 (-6.9601, 54.1141) -> (-6.9601, 53.5333)
  line L44 (-6.923, 53.5333) -> (-5.8923, 56.5833)
  line L45 (-5.8923, 56.5833) -> (-5.0569, 56.5833)
  line L46 (-5.0569, 56.5833) -> (-4.0262, 53.5333)
  line L47 (-4.0262, 53.5333) -> (-4.8147, 53.5333)
  line L48 (-4.8147, 53.5333) -> (-5.005, 54.1561)
  line L49 (-5.005, 54.1561) -> (-5.964, 54.1561)
  line L50 (-5.964, 54.1561) -> (-6.1568, 53.5333)
  line L51 (-6.1568, 53.5333) -> (-6.923, 53.5333)
  line L52 (-5.1731, 54.7098) -> (-5.4845, 55.7182)
  line L53 (-5.4845, 55.7182) -> (-5.7984, 54.7098)
  line L54 (-5.7984, 54.7098) -> (-5.1731, 54.7098)
  spline S23 degree 2 poles (-1.2852, 54.4676) (-1.2852, 54.2402) (-1.4582, 53.8966) (-1.6016, 53.7829) knots 0 0 0 1 2 2 2
  spline S24 degree 2 poles (-1.6016, 53.7829) (-1.7746, 53.647) (-2.1849, 53.5333) (-2.5037, 53.5333) knots 0 0 0 1 2 2 2
  line L55 (-2.5037, 53.5333) -> (-3.7222, 53.5333)
  line L56 (-3.7222, 53.5333) -> (-3.7222, 56.5833)
  line L57 (-3.7222, 56.5833) -> (-2.6471, 56.5833)
  spline S25 degree 2 poles (-2.6471, 56.5833) (-2.3109, 56.5833) (-1.9649, 56.5314) (-1.8141, 56.4498) knots 0 0 0 1 2 2 2
  spline S26 degree 2 poles (-1.8141, 56.4498) (-1.6485, 56.3633) (-1.4879, 56.0667) (-1.4879, 55.8739) knots 0 0 0 1 2 2 2
  spline S27 degree 2 poles (-1.4879, 55.8739) (-1.4879, 55.6515) (-1.7103, 55.303) (-1.908, 55.2214) knots 0 0 0 1 2 2 2
  line L58 (-1.908, 55.2214) -> (-1.908, 55.2066)
  spline S28 degree 2 poles (-1.908, 55.2066) (-1.6238, 55.1473) (-1.2852, 54.779) (-1.2852, 54.4676) knots 0 0 0 1 2 2 2
  spline S29 degree 2 poles (-2.0761, 54.4799) (-2.0761, 54.6233) (-2.1898, 54.7839) (-2.3035, 54.8259) knots 0 0 0 1 2 2 2
  spline S30 degree 2 poles (-2.3035, 54.8259) (-2.3727, 54.8531) (-2.6174, 54.8581) (-2.8201, 54.8581) knots 0 0 0 1 2 2 2
  line L59 (-2.8201, 54.8581) -> (-2.961, 54.8581)
  line L60 (-2.961, 54.8581) -> (-2.961, 54.0894)
  line L61 (-2.961, 54.0894) -> (-2.9189, 54.0894)
  spline S31 degree 2 poles (-2.9189, 54.0894) (-2.6224, 54.0894) (-2.395, 54.0968) (-2.2763, 54.1487) knots 0 0 0 1 2 2 2
  spline S32 degree 2 poles (-2.2763, 54.1487) (-2.1725, 54.1957) (-2.0761, 54.3687) (-2.0761, 54.4799) knots 0 0 0 1 2 2 2
  spline S33 degree 2 poles (-2.2664, 55.7231) (-2.2664, 55.7973) (-2.3431, 55.953) (-2.4221, 55.9876) knots 0 0 0 1 2 2 2
  spline S34 degree 2 poles (-2.4221, 55.9876) (-2.4963, 56.0222) (-2.7039, 56.0272) (-2.9091, 56.0272) knots 0 0 0 1 2 2 2
  line L62 (-2.9091, 56.0272) -> (-2.961, 56.0272)
  line L63 (-2.961, 56.0272) -> (-2.961, 55.3796)
  line L64 (-2.961, 55.3796) -> (-2.8646, 55.3796)
  spline S35 degree 2 poles (-2.8646, 55.3796) (-2.6693, 55.3796) (-2.5111, 55.387) (-2.4271, 55.4265) knots 0 0 0 1 2 2 2
  spline S36 degree 2 poles (-2.4271, 55.4265) (-2.3356, 55.471) (-2.2664, 55.6218) (-2.2664, 55.7231) knots 0 0 0 1 2 2 2
  spline S37 degree 2 poles (-20.711, 49.5447) (-20.711, 49.3049) (-20.8742, 48.8996) (-21.0348, 48.7538) knots 0 0 0 1 2 2 2
  spline S38 degree 2 poles (-21.0348, 48.7538) (-21.1955, 48.6079) (-21.6354, 48.4473) (-21.9567, 48.4473) knots 0 0 0 1 2 2 2
  spline S39 degree 2 poles (-21.9567, 48.4473) (-22.2978, 48.4497) (-22.7872, 48.561) (-22.9479, 48.6326) knots 0 0 0 1 2 2 2
  line L65 (-22.9479, 48.6326) -> (-22.9479, 49.2975)
  line L66 (-22.9479, 49.2975) -> (-22.8787, 49.2975)
  spline S40 degree 2 poles (-22.8787, 49.2975) (-22.8193, 49.2654) (-22.676, 49.1813) (-22.5598, 49.1369) knots 0 0 0 1 2 2 2
  spline S41 degree 2 poles (-22.5598, 49.1369) (-22.4511, 49.0948) (-22.2261, 49.038) (-22.0902, 49.038) knots 0 0 0 1 2 2 2
  spline S42 degree 2 poles (-22.0902, 49.038) (-21.9716, 49.038) (-21.6947, 49.0973) (-21.6107, 49.1764) knots 0 0 0 1 2 2 2
  spline S43 degree 2 poles (-21.6107, 49.1764) (-21.5489, 49.2382) (-21.4797, 49.389) (-21.4797, 49.515) knots 0 0 0 1 2 2 2
  spline S44 degree 2 poles (-21.4797, 49.515) (-21.4797, 49.6238) (-21.5687, 49.777) (-21.6404, 49.824) knots 0 0 0 1 2 2 2
  spline S45 degree 2 poles (-21.6404, 49.824) (-21.7442, 49.8932) (-22.0408, 49.9327) (-22.147, 49.9327) knots 0 0 0 1 2 2 2
  spline S46 degree 2 poles (-22.147, 49.9327) (-22.3151, 49.9327) (-22.634, 49.8783) (-22.7501, 49.8487) knots 0 0 0 1 2 2 2
  line L67 (-22.7501, 49.8487) -> (-22.8169, 49.8487)
  line L68 (-22.8169, 49.8487) -> (-22.8169, 51.5615)
  line L69 (-22.8169, 51.5615) -> (-20.7951, 51.5615)
  line L70 (-20.7951, 51.5615) -> (-20.7951, 50.9856)
  line L71 (-20.7951, 50.9856) -> (-22.0927, 50.9856)
  line L72 (-22.0927, 50.9856) -> (-22.0927, 50.479)
  spline S47 degree 2 poles (-22.0927, 50.479) (-22.0309, 50.4839) (-21.8603, 50.4888) (-21.8134, 50.4888) knots 0 0 0 1 2 2 2
  spline S48 degree 2 poles (-21.8134, 50.4888) (-21.5934, 50.4888) (-21.2227, 50.3999) (-21.0768, 50.3084) knots 0 0 0 1 2 2 2
  spline S49 degree 2 poles (-21.0768, 50.3084) (-20.9038, 50.1947) (-20.711, 49.8166) (-20.711, 49.5447) knots 0 0 0 1 2 2 2
  line L73 (-18.4767, 51.6975) -> (-19.6902, 47.8491)
  line L74 (-19.6902, 47.8491) -> (-20.2785, 47.8491)
  line L75 (-20.2785, 47.8491) -> (-19.0674, 51.6975)
  line L76 (-19.0674, 51.6975) -> (-18.4767, 51.6975)
  line L77 (-15.5502, 48.5115) -> (-17.792, 48.5115)
  line L78 (-17.792, 48.5115) -> (-17.792, 49.0083)
  spline S50 degree 2 poles (-17.792, 49.0083) (-17.5078, 49.2357) (-17.053, 49.6361) (-16.8825, 49.8166) knots 0 0 0 1 2 2 2
  spline S51 degree 2 poles (-16.8825, 49.8166) (-16.6575, 50.0514) (-16.4573, 50.4097) (-16.4573, 50.5976) knots 0 0 0 1 2 2 2
  spline S52 degree 2 poles (-16.4573, 50.5976) (-16.4573, 50.8102) (-16.7119, 51.0375) (-16.9393, 51.0375) knots 0 0 0 1 2 2 2
  spline S53 degree 2 poles (-16.9393, 51.0375) (-17.0555, 51.0375) (-17.2631, 50.9807) (-17.3694, 50.9362) knots 0 0 0 1 2 2 2
  spline S54 degree 2 poles (-17.3694, 50.9362) (-17.4732, 50.8892) (-17.6215, 50.7904) (-17.6586, 50.7657) knots 0 0 0 1 2 2 2
  line L79 (-17.6586, 50.7657) -> (-17.7179, 50.7657)
  line L80 (-17.7179, 50.7657) -> (-17.7179, 51.4305)
  spline S55 degree 2 poles (-17.7179, 51.4305) (-17.5893, 51.4923) (-17.0406, 51.6208) (-16.7861, 51.6208) knots 0 0 0 1 2 2 2
  spline S56 degree 2 poles (-16.7861, 51.6208) (-16.2423, 51.6208) (-15.6837, 51.1364) (-15.6837, 50.6989) knots 0 0 0 1 2 2 2
  spline S57 degree 2 poles (-15.6837, 50.6989) (-15.6837, 50.4295) (-15.9383, 49.9105) (-16.2324, 49.6139) knots 0 0 0 1 2 2 2
  spline S58 degree 2 poles (-16.2324, 49.6139) (-16.4178, 49.431) (-16.7663, 49.1467) (-16.8429, 49.0874) knots 0 0 0 1 2 2 2
  line L81 (-16.8429, 49.0874) -> (-15.5502, 49.0874)
  line L82 (-15.5502, 49.0874) -> (-15.5502, 48.5115)
  line L83 (-13.0143, 48.5115) -> (-15.0287, 48.5115)
  line L84 (-15.0287, 48.5115) -> (-15.0287, 49.0429)
  line L85 (-15.0287, 49.0429) -> (-14.3861, 49.0429)
  line L86 (-14.3861, 49.0429) -> (-14.3861, 50.6569)
  line L87 (-14.3861, 50.6569) -> (-15.0287, 50.6569)
  line L88 (-15.0287, 50.6569) -> (-15.0287, 51.1537)
  spline S59 degree 2 poles (-15.0287, 51.1537) (-14.8878, 51.1537) (-14.6086, 51.1908) (-14.5245, 51.2303) knots 0 0 0 1 2 2 2
  spline S60 degree 2 poles (-14.5245, 51.2303) (-14.4281, 51.2798) (-14.3194, 51.4454) (-14.3095, 51.5689) knots 0 0 0 1 2 2 2
  line L89 (-14.3095, 51.5689) -> (-13.6421, 51.5689)
  line L90 (-13.6421, 51.5689) -> (-13.6421, 49.0429)
  line L91 (-13.6421, 49.0429) -> (-13.0143, 49.0429)
  line L92 (-13.0143, 49.0429) -> (-13.0143, 48.5115)
  line L93 (-10.7133, 51.6975) -> (-11.9268, 47.8491)
  line L94 (-11.9268, 47.8491) -> (-12.5151, 47.8491)
  line L95 (-12.5151, 47.8491) -> (-11.304, 51.6975)
  line L96 (-11.304, 51.6975) -> (-10.7133, 51.6975)
  line L97 (-7.7868, 48.5115) -> (-10.0286, 48.5115)
  line L98 (-10.0286, 48.5115) -> (-10.0286, 49.0083)
  spline S61 degree 2 poles (-10.0286, 49.0083) (-9.7444, 49.2357) (-9.2896, 49.6361) (-9.119, 49.8166) knots 0 0 0 1 2 2 2
  spline S62 degree 2 poles (-9.119, 49.8166) (-8.8941, 50.0514) (-8.6939, 50.4097) (-8.6939, 50.5976) knots 0 0 0 1 2 2 2
  spline S63 degree 2 poles (-8.6939, 50.5976) (-8.6939, 50.8102) (-8.9485, 51.0375) (-9.1759, 51.0375) knots 0 0 0 1 2 2 2
  spline S64 degree 2 poles (-9.1759, 51.0375) (-9.2921, 51.0375) (-9.4997, 50.9807) (-9.606, 50.9362) knots 0 0 0 1 2 2 2
  spline S65 degree 2 poles (-9.606, 50.9362) (-9.7098, 50.8892) (-9.8581, 50.7904) (-9.8951, 50.7657) knots 0 0 0 1 2 2 2
  line L99 (-9.8951, 50.7657) -> (-9.9545, 50.7657)
  line L100 (-9.9545, 50.7657) -> (-9.9545, 51.4305)
  spline S66 degree 2 poles (-9.9545, 51.4305) (-9.8259, 51.4923) (-9.2772, 51.6208) (-9.0227, 51.6208) knots 0 0 0 1 2 2 2
  spline S67 degree 2 poles (-9.0227, 51.6208) (-8.4789, 51.6208) (-7.9203, 51.1364) (-7.9203, 50.6989) knots 0 0 0 1 2 2 2
  spline S68 degree 2 poles (-7.9203, 50.6989) (-7.9203, 50.4295) (-8.1749, 49.9105) (-8.469, 49.6139) knots 0 0 0 1 2 2 2
  spline S69 degree 2 poles (-8.469, 49.6139) (-8.6544, 49.431) (-9.0029, 49.1467) (-9.0795, 49.0874) knots 0 0 0 1 2 2 2
  line L101 (-9.0795, 49.0874) -> (-7.7868, 49.0874)
  line L102 (-7.7868, 49.0874) -> (-7.7868, 48.5115)
  spline S70 degree 2 poles (-5.1545, 50.0365) (-5.1545, 49.6411) (-5.2806, 49.0479) (-5.4215, 48.8477) knots 0 0 0 1 2 2 2
  spline S71 degree 2 poles (-5.4215, 48.8477) (-5.5599, 48.6499) (-6.0073, 48.4473) (-6.3286, 48.4473) knots 0 0 0 1 2 2 2
  spline S72 degree 2 poles (-6.3286, 48.4473) (-6.6524, 48.4473) (-7.0972, 48.6499) (-7.2381, 48.8526) knots 0 0 0 1 2 2 2
  spline S73 degree 2 poles (-7.2381, 48.8526) (-7.379, 49.0528) (-7.5051, 49.6411) (-7.5051, 50.0365) knots 0 0 0 1 2 2 2
  spline S74 degree 2 poles (-7.5051, 50.0365) (-7.5051, 50.4419) (-7.379, 51.0153) (-7.2357, 51.2229) knots 0 0 0 1 2 2 2
  spline S75 degree 2 poles (-7.2357, 51.2229) (-7.0923, 51.4256) (-6.64, 51.6233) (-6.3286, 51.6233) knots 0 0 0 1 2 2 2
  spline S76 degree 2 poles (-6.3286, 51.6233) (-5.9998, 51.6233) (-5.5599, 51.4157) (-5.419, 51.2106) knots 0 0 0 1 2 2 2
  spline S77 degree 2 poles (-5.419, 51.2106) (-5.2806, 51.0104) (-5.1545, 50.4196) (-5.1545, 50.0365) knots 0 0 0 1 2 2 2
  spline S78 degree 2 poles (-5.9232, 50.0365) (-5.9232, 50.6025) (-6.1086, 51.0598) (-6.3286, 51.0598) knots 0 0 0 1 2 2 2
  spline S79 degree 2 poles (-6.3286, 51.0598) (-6.5485, 51.0598) (-6.7364, 50.6025) (-6.7364, 50.0341) knots 0 0 0 1 2 2 2
  spline S80 degree 2 poles (-6.7364, 50.0341) (-6.7364, 49.4755) (-6.5485, 49.0108) (-6.3286, 49.0108) knots 0 0 0 1 2 2 2
  spline S81 degree 2 poles (-6.3286, 49.0108) (-6.1111, 49.0108) (-5.9232, 49.4755) (-5.9232, 50.0365) knots 0 0 0 1 2 2 2
  line L103 (-2.4432, 48.5115) -> (-4.6849, 48.5115)
  line L104 (-4.6849, 48.5115) -> (-4.6849, 49.0083)
  spline S82 degree 2 poles (-4.6849, 49.0083) (-4.4007, 49.2357) (-3.9459, 49.6361) (-3.7754, 49.8166) knots 0 0 0 1 2 2 2
  spline S83 degree 2 poles (-3.7754, 49.8166) (-3.5504, 50.0514) (-3.3502, 50.4097) (-3.3502, 50.5976) knots 0 0 0 1 2 2 2
  spline S84 degree 2 poles (-3.3502, 50.5976) (-3.3502, 50.8102) (-3.6048, 51.0375) (-3.8322, 51.0375) knots 0 0 0 1 2 2 2
  spline S85 degree 2 poles (-3.8322, 51.0375) (-3.9484, 51.0375) (-4.156, 50.9807) (-4.2623, 50.9362) knots 0 0 0 1 2 2 2
  spline S86 degree 2 poles (-4.2623, 50.9362) (-4.3661, 50.8892) (-4.5144, 50.7904) (-4.5515, 50.7657) knots 0 0 0 1 2 2 2
  line L105 (-4.5515, 50.7657) -> (-4.6108, 50.7657)
  line L106 (-4.6108, 50.7657) -> (-4.6108, 51.4305)
  spline S87 degree 2 poles (-4.6108, 51.4305) (-4.4823, 51.4923) (-3.9336, 51.6208) (-3.679, 51.6208) knots 0 0 0 1 2 2 2
  spline S88 degree 2 poles (-3.679, 51.6208) (-3.1352, 51.6208) (-2.5766, 51.1364) (-2.5766, 50.6989) knots 0 0 0 1 2 2 2
  spline S89 degree 2 poles (-2.5766, 50.6989) (-2.5766, 50.4295) (-2.8312, 49.9105) (-3.1253, 49.6139) knots 0 0 0 1 2 2 2
  spline S90 degree 2 poles (-3.1253, 49.6139) (-3.3107, 49.431) (-3.6592, 49.1467) (-3.7358, 49.0874) knots 0 0 0 1 2 2 2
  line L107 (-3.7358, 49.0874) -> (-2.4432, 49.0874)
  line L108 (-2.4432, 49.0874) -> (-2.4432, 48.5115)
  spline S91 degree 2 poles (0.2114, 49.5496) (0.2114, 49.0676) (-0.3991, 48.4473) (-0.933, 48.4473) knots 0 0 0 1 2 2 2
  spline S92 degree 2 poles (-0.933, 48.4473) (-1.1999, 48.4473) (-1.6176, 48.6005) (-1.7635, 48.7513) knots 0 0 0 1 2 2 2
  spline S93 degree 2 poles (-1.7635, 48.7513) (-1.9365, 48.9268) (-2.1218, 49.4829) (-2.1218, 49.8709) knots 0 0 0 1 2 2 2
  spline S94 degree 2 poles (-2.1218, 49.8709) (-2.1218, 50.2713) (-1.9488, 50.8942) (-1.7536, 51.1339) knots 0 0 0 1 2 2 2
  spline S95 degree 2 poles (-1.7536, 51.1339) (-1.5682, 51.3613) (-0.9651, 51.6184) (-0.5524, 51.6184) knots 0 0 0 1 2 2 2
  spline S96 degree 2 poles (-0.5524, 51.6184) (-0.4016, 51.6184) (-0.1, 51.5788) (-0.0457, 51.5665) knots 0 0 0 1 2 2 2
  line L109 (-0.0457, 51.5665) -> (-0.0457, 50.9683)
  line L110 (-0.0457, 50.9683) -> (-0.1, 50.9683)
  spline S97 degree 2 poles (-0.1, 50.9683) (-0.1544, 50.9955) (-0.4016, 51.0623) (-0.5598, 51.0623) knots 0 0 0 1 2 2 2
  spline S98 degree 2 poles (-0.5598, 51.0623) (-0.9182, 51.0623) (-1.3087, 50.6841) (-1.3556, 50.3331) knots 0 0 0 1 2 2 2
  spline S99 degree 2 poles (-1.3556, 50.3331) (-1.2049, 50.4295) (-0.8959, 50.5432) (-0.7007, 50.5432) knots 0 0 0 1 2 2 2
  spline S100 degree 2 poles (-0.7007, 50.5432) (-0.5351, 50.5432) (-0.2459, 50.4542) (-0.1346, 50.3702) knots 0 0 0 1 2 2 2
  spline S101 degree 2 poles (-0.1346, 50.3702) (0.0235, 50.2491) (0.2114, 49.8561) (0.2114, 49.5496) knots 0 0 0 1 2 2 2
  spline S102 degree 2 poles (-0.6809, 49.0899) (-0.6216, 49.164) (-0.5573, 49.3371) (-0.5573, 49.5125) knots 0 0 0 1 2 2 2
  spline S103 degree 2 poles (-0.5573, 49.5125) (-0.5573, 49.6608) (-0.6314, 49.8536) (-0.6982, 49.9105) knots 0 0 0 1 2 2 2
  spline S104 degree 2 poles (-0.6982, 49.9105) (-0.7674, 49.9698) (-0.9379, 50.0118) (-1.0343, 50.0118) knots 0 0 0 1 2 2 2
  spline S105 degree 2 poles (-1.0343, 50.0118) (-1.1159, 50.0118) (-1.284, 49.9698) (-1.3581, 49.9401) knots 0 0 0 1 2 2 2
  spline S106 degree 2 poles (-1.3581, 49.9401) (-1.3581, 49.9204) (-1.3631, 49.8264) (-1.3631, 49.7548) knots 0 0 0 1 2 2 2
  spline S107 degree 2 poles (-1.3631, 49.7548) (-1.3631, 49.4903) (-1.2716, 49.1715) (-1.1999, 49.0899) knots 0 0 0 1 2 2 2
  spline S108 degree 2 poles (-1.1999, 49.0899) (-1.148, 49.0232) (-1.0096, 48.9663) (-0.9355, 48.9663) knots 0 0 0 1 2 2 2
  spline S109 degree 2 poles (-0.9355, 48.9663) (-0.8737, 48.9663) (-0.7303, 49.0281) (-0.6809, 49.0899) knots 0 0 0 1 2 2 2
  point P0 (0, 0)
  dimension "d0" = 19
  dimension "d2" = 19
  dimension "d4" = 19
  dimension "d53" = 19
  dimension "d144" = 28
  dimension "d145" = 28
  dimension "d149" = 28
  dimension "d150" = 28
  dimension "d154" = 30
  dimension "d158" = 30
  dimension "d162" = 30
  dimension "d163" = 30
  dimension "d291" = 19
  dimension "d292" = 28
  dimension "d293" = 30
  dimension "d294" = 19
  dimension "d295" = 19
  dimension "d296" = 28
  dimension "d297" = 30
  dimension "d298" = 28
  dimension "d299" = 30
  constraints: 2 other
extrude "Extrusion35" add sketch "Sketch39" along normal blind 2
body "Solid1"
